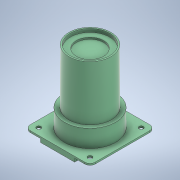
# Autodesk Inventor part: camera
Saved by Autodesk Inventor 2021 (Build 250183000, 183)
## iProperties
Created: 2021-02-15
Part Number: camera
Material: Generic
Document SubType Name: Modeling
Designer: lobato
Density: 1 g/cm^3
Appearance: Default
Author: lobato
Autodesk Inventor part; units mm, degrees
ref_plane "YZ Plane" through (0, 0, 0) normal (1, 0, 0) x (0, 1, 0)
ref_plane "XZ Plane" through (0, 0, 0) normal (0, 1, 0) x (-1, 0, 0)
ref_plane "XY Plane" through (0, 0, 0) normal (0, 0, 1) x (1, 0, 0)
sketch "Sketch1" plane through (0, 0, 0) normal (0, 1, 0) x (-1, 0, 0)
  line L0 (19, 19) -> (-19, 19)
  line L1 (-19, 19) -> (-19, -19)
  line L2 (-19, -19) -> (19, -19)
  line L3 (19, -19) -> (19, 19)
  line L4 (19, 19) -> (-19, -19) construction
  line L5 (-19, 19) -> (19, -19) construction
  line L6 (15, 15) -> (-15, 15) construction
  line L7 (-15, 15) -> (-15, -15) construction
  line L8 (-15, -15) -> (15, -15) construction
  line L9 (15, -15) -> (15, 15) construction
  line L10 (15, 15) -> (-15, -15) construction
  line L11 (-15, 15) -> (15, -15) construction
  circle A0 centre (15, 15) radius 1.25
  circle A1 centre (15, -15) radius 1.25
  circle A2 centre (-15, -15) radius 1.25
  circle A3 centre (-15, 15) radius 1.25
  point P0 (0, 0)
  dimension "d0" = 38
  dimension "d1" = 38
  dimension "d2" = 30
  dimension "d3" = 30
  dimension "d4" = 2.5
  dimension "d5" = 2.5
  dimension "d6" = 2.5
  dimension "d7" = 2.5
  constraints: 24 end point, 4 centre point, 4 coincident, 4 midpoint, 4 parallel, 2 horizontal, 2 perpendicular
  measures "d0" distance of L2.end L1.end
  measures "d1" distance of L1.end L0.end
  measures "d2" distance of L8.end L7.end
  measures "d3" distance of L7.end L6.end
  measures "d4" diameter of A0
  measures "d5" diameter of A1
  measures "d6" diameter of A2
  measures "d7" diameter of A3
extrude "Extrusion1" add sketch "Sketch1" along normal blind 1
fillet "Fillet1" radius 3 4 edges at (19, 0.5, 19) (19, 0.5, -19) (-19, 0.5, -19) (-19, 0.5, 19)
sketch "Sketch2" plane through (0, 0, 0) normal (1, 0, 0) x (0, 1, 0)
  line L0 (43.1895, 0) -> (0.9392, 0)
  line L1 (1, 16) -> (1, -16) construction
  line L2 (0, 16) -> (0, -16) projected
  line L3 (0.9392, 0) -> (1, -14.9999)
  line L4 (1, -16) -> (1, 16) projected
  line L5 (1, -14.9999) -> (11.1999, -14.9585)
  line L6 (11.1999, -14.9585) -> (11.1898, -12.4586)
  line L7 (11.1898, -12.4586) -> (43.1895, -12.3289)
  line L8 (43.1895, -12.3289) -> (43.1895, 0)
  point P0 (0, 0)
  dimension "d16" = 15
  dimension "d17" = 10.2
  dimension "d18" = 2.5
  dimension "d19" = 32
  constraints: 12 end point, 5 perpendicular, 1 point on line
  measures "d16" distance of L0.end L3.end
  measures "d17" distance of L3.end L5.end
  measures "d18" distance of L5.end L6.end
  measures "d19" distance of L6.end L7.end
revolve "Revolution1" add sketch "Sketch2" angle 360 about axis through (0, 43.1895, 0) along (0, -1, 0)
sketch "Sketch3" plane through (0, 43.1895, 0) normal (0, 1, 0) x (1, 0, 0)
  circle A0 centre (0, 0) radius 11.5
  dimension "d20" = 23
  constraints: 1 centre point, 1 coincident
  measures "d20" diameter of A0
extrude "Extrusion2" cut sketch "Sketch3" against normal blind 2
sketch "Sketch4" plane through (0, 41.1895, 0) normal (0, 1, 0) x (1, 0, 0)
  circle A0 centre (0, 0) radius 8
  dimension "d23" = 16
  constraints: 1 centre point, 1 coincident
  measures "d23" diameter of A0
extrude "Extrusion3" cut sketch "Sketch4" against normal blind 1
sketch "Sketch5" plane through (0, 0, 0) normal (0, -1, 0) x (1, 0, 0)
  circle A0 centre (-12, 0) radius 2.5
  line L0 (-19, -16) -> (-19, 16) projected
  circle A1 centre (12, 0) radius 2.5
  line L1 (19, 16) -> (19, -16) projected
  point P0 (0, 0)
  dimension "d26" = 5
  dimension "d27" = 7
  dimension "d28" = 5
  dimension "d29" = 7
  constraints: 2 centre point
  measures "d26" diameter of A0
  measures "d27" distance from line of L0 A0.centre
  measures "d28" diameter of A1
  measures "d29" distance from line of L1 A1.centre
extrude "Extrusion4" add sketch "Sketch5" along normal blind 3
sketch "Sketch6" plane through (0, 0, 0) normal (0, -1, 0) x (1, 0, 0)
  line L0 (-16, 19) -> (16, 19) projected
  line L1 (-10, 13.5) -> (10, 13.5)
  line L2 (10, 13.5) -> (10, 19)
  line L3 (10, 19) -> (-10, 19)
  line L4 (-10, 19) -> (-10, 13.5)
  line L5 (-10, 13.5) -> (10, 19) construction
  line L6 (10, 13.5) -> (-10, 19) construction
  point P0 (0, 0)
  point P1 (0, 16.25)
  dimension "d32" = 20
  dimension "d33" = 5.5
  constraints: 12 end point, 2 midpoint, 2 parallel, 1 horizontal, 1 perpendicular, 1 point on line
  measures "d32" distance of L3.end L2.end
  measures "d33" distance between parallel lines of L1 L0
extrude "Extrusion5" add sketch "Sketch6" along normal blind 2
body "Solid1"
